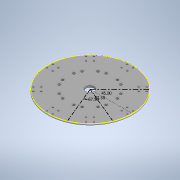
# Autodesk Inventor part: MainDisk1
Saved by Autodesk Inventor 2022.1 (Build 261234020, 234B)
## iProperties
Created: 2021-11-14
Part Number: MainDisk1
Material: Generic
Document SubType Name: Modeling
Designer: Alexander
Density: 1 g/cm^3
Appearance: Default
Author: Alexander
Autodesk Inventor part; units mm, degrees
ref_plane "YZ Plane" through (0, 0, 0) normal (1, 0, 0) x (0, 1, 0)
ref_plane "XZ Plane" through (0, 0, 0) normal (0, 1, 0) x (-1, 0, 0)
ref_plane "XY Plane" through (0, 0, 0) normal (0, 0, 1) x (1, 0, 0)
sketch "Sketch1" plane through (0, 0, 0) normal (0, 1, 0) x (-1, 0, 0)
  circle A0 centre (0, 0) radius 150
  circle A1 centre (143, 10) radius 2.25
  line L0 (18.6053, 16.2989) -> (18.6053, 8.3379)
  line L1 (18.6053, 8.3379) -> (11.4784, 8.3379)
  circle A2 centre (143, -10) radius 2.25
  circle A3 centre (123, 10) radius 2.25
  circle A4 centre (123, -10) radius 2.25
  line L2 (114.6014, 0) -> (140.75, 0)
  line L3 (150, 0) -> (150, 14.1456)
  circle A5 centre (94.0452, 79.9031) radius 2.25
  circle A6 centre (108.1873, 94.0452) radius 2.25
  circle A7 centre (94.0452, 108.1873) radius 2.25
  circle A8 centre (79.9031, 94.0452) radius 2.25
  circle A9 centre (10, 123) radius 2.25
  circle A10 centre (10, 143) radius 2.25
  circle A11 centre (-10, 143) radius 2.25
  circle A12 centre (-10, 123) radius 2.25
  circle A13 centre (-79.9031, 94.0452) radius 2.25
  circle A14 centre (-94.0452, 108.1873) radius 2.25
  circle A15 centre (-108.1873, 94.0452) radius 2.25
  circle A16 centre (-94.0452, 79.9031) radius 2.25
  circle A17 centre (-123, 10) radius 2.25
  circle A18 centre (-143, 10) radius 2.25
  circle A19 centre (-143, -10) radius 2.25
  circle A20 centre (-123, -10) radius 2.25
  circle A21 centre (-94.0452, -79.9031) radius 2.25
  circle A22 centre (-108.1873, -94.0452) radius 2.25
  circle A23 centre (-94.0452, -108.1873) radius 2.25
  circle A24 centre (-79.9031, -94.0452) radius 2.25
  circle A25 centre (-10, -123) radius 2.25
  circle A26 centre (-10, -143) radius 2.25
  circle A27 centre (10, -143) radius 2.25
  circle A28 centre (10, -123) radius 2.25
  circle A29 centre (79.9031, -94.0452) radius 2.25
  circle A30 centre (94.0452, -108.1873) radius 2.25
  circle A31 centre (108.1873, -94.0452) radius 2.25
  circle A32 centre (94.0452, -79.9031) radius 2.25
  circle A33 centre (0, 0) radius 15
  circle A34 centre (77.6531, -20) radius 3.75
  circle A35 centre (77.6531, 20) radius 3.75
  circle A36 centre (69.0511, 40.7669) radius 3.75
  circle A37 centre (40.7669, 69.0511) radius 3.75
  circle A38 centre (20, 77.6531) radius 3.75
  circle A39 centre (-20, 77.6531) radius 3.75
  circle A40 centre (-40.7669, 69.0511) radius 3.75
  circle A41 centre (-69.0511, 40.7669) radius 3.75
  circle A42 centre (-77.6531, 20) radius 3.75
  circle A43 centre (-77.6531, -20) radius 3.75
  circle A44 centre (-69.0511, -40.7669) radius 3.75
  circle A45 centre (-40.7669, -69.0511) radius 3.75
  circle A46 centre (-20, -77.6531) radius 3.75
  circle A47 centre (20, -77.6531) radius 3.75
  circle A48 centre (40.7669, -69.0511) radius 3.75
  circle A49 centre (69.0511, -40.7669) radius 3.75
  dimension "d0" = 300
  dimension "d3" = 4.5
  dimension "d7" = 20
  dimension "d10" = 20
  dimension "d13" = 20
  dimension "d14" = 14
  dimension "d17" = 360
  dimension "d21" = 30
  dimension "d22" = 7.5
  dimension "d23" = 40
  dimension "d26" = 360
  constraints: 49 centre point, 8 end point, 3 vertical, 2 coincident, 2 horizontal, 1 horizontal alignment, 1 perpendicular, 1 symmetric about line, 107 other
  measures "d3" diameter of A1
  measures "d7" distance of A1.centre A2.centre
  measures "d10" distance of A1.centre A3.centre
  measures "d13" diameter of A3.centre L2
  measures "d14" diameter of A1.centre L3
  measures "d21" diameter of A33
  measures "d22" diameter of A34
  measures "d23" diameter of A34.centre L2
extrude "Extrusion2" add sketch "Sketch1" along normal blind 5
sketch "Sketch2" plane through (0, 5, 0) normal (0, 1, 0) x (1, 0, 0)
  line L0 (0, 0) -> (106.066, 106.066)
  circle A0 centre (0, 0) radius 150 projected
  line L1 (0, 0) -> (150, 0) construction
  line L2 (0, 0) -> (138.5819, -57.4025)
  line L3 (0, 0) -> (150, 0) construction
  line L4 (0, 0) -> (57.4025, -138.5819)
  line L5 (0, 0) -> (150, 0) construction
  dimension "d28" = 45
  dimension "d29" = 22.5
  dimension "d30" = 67.5
  constraints: 12 end point, 3 equal length, 3 horizontal, 3 point on circle
  measures "d28" angle of L1 L0
  measures "d29" angle of L2 L3
  measures "d30" angle of L4 L5
body "Solid2"
